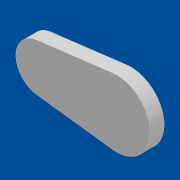
# Autodesk Inventor part: 111-base template
Saved by Autodesk Inventor 2018 (Build 220112000, 112)
## iProperties
Created: 2019-11-07
Part Number: 111-base template
Material: Generic
Document SubType Name: Modeling
Designer: Bunny320
Density: 1 g/cm^3
Appearance: Default
Author: Bunny320
Autodesk Inventor part; units mm, degrees
ref_plane "YZ Plane" through (0, 0, 0) normal (1, 0, 0) x (0, 1, 0)
ref_plane "XZ Plane" through (0, 0, 0) normal (0, 1, 0) x (-1, 0, 0)
ref_plane "XY Plane" through (0, 0, 0) normal (0, 0, 1) x (1, 0, 0)
sketch "Sketch2" plane through (0, 0, 0) normal (0, 1, 0) x (-1, 0, 0)
  circle A0 centre (0, 0) radius 40
  circle A1 centre (-141.8, 0) radius 57.5
  line L0 (4.9365, -39.6942) -> (-134.7037, -57.0604)
  line L1 (4.9365, 39.6942) -> (-134.7037, 57.0604)
  dimension "d5" = 141.8
  dimension "d6" = 80
  dimension "d7" = 115
  constraints: 4 end point, 4 point on circle, 4 tangent, 2 centre point, 1 coincident, 1 horizontal alignment
  measures "d5" distance of A1.centre point (0, 0)
  measures "d6" diameter of A0
  measures "d7" diameter of A1
extrude "Extrusion2" add sketch "Sketch2" along normal blind 4
sketch "Sketch14" plane through (0, 0, 0) normal (0, 1, 0) x (-1, 0, 0)
  arc A0 (4.9365, -39.6942) -> (4.9365, 39.6942) centre (0, 0) ccw projected
  arc A1 (5.4302, -43.6636) -> (5.4302, 43.6636) centre (0, 0) ccw
  arc A2 (-134.7037, 57.0604) -> (-134.7037, -57.0604) centre (-141.8, 0) ccw projected
  arc A3 (-134.2101, 61.0299) -> (-134.2101, -61.0299) centre (-141.8, 0) ccw
  line L0 (5.4302, -43.6636) -> (-134.2101, -61.0299)
  line L1 (-134.2101, 61.0299) -> (5.4302, 43.6636)
  line L2 (-134.7037, -57.0604) -> (4.9365, -39.6942)
  arc A4 (4.9365, -39.6942) -> (4.9365, 39.6942) centre (0, 0) ccw
  line L3 (4.9365, 39.6942) -> (-134.7037, 57.0604)
  arc A5 (-134.7037, 57.0604) -> (-134.7037, -57.0604) centre (-141.8, 0) ccw
  dimension "d53" = 4
  dimension "d54" = 4
  dimension "d55" = 4
  constraints: 8 end point, 8 point on circle, 4 centre point, 4 tangent, 2 coincident, 3 other
  measures "d53" radial gap between concentric circles of A0 A1
  measures "d54" radial gap between concentric circles of A2 A3
  measures "d55" distance between parallel lines of L2 L0
extrude "Extrusion11" add sketch "Sketch14" along normal blind 26
sketch "Sketch27" plane through (0, 4, 0) normal (0, 1, 0) x (1, 0, 0)
  line L0 (-40, 4) -> (-36, 4)
  line L1 (-36, 4) -> (-36, -4)
  line L2 (-36, -4) -> (-40, -4)
  line L3 (-40, -4) -> (-40, 4)
  line L4 (-40, 4) -> (-36, -4) construction
  line L5 (-36, 4) -> (-40, -4) construction
  arc A0 (-4.9365, 39.6942) -> (-4.9365, -39.6942) centre (0, 0) ccw projected
  line L6 (-4.9365, 39.6942) -> (134.7037, 57.0604) projected
  arc A1 (134.7037, -57.0604) -> (134.7037, 57.0604) centre (141.8, 0) ccw projected
  line L7 (195.3, 4) -> (199.3, 4)
  line L8 (199.3, 4) -> (199.3, -4)
  line L9 (199.3, -4) -> (195.3, -4)
  line L10 (195.3, -4) -> (195.3, 4)
  line L11 (195.3, 4) -> (199.3, -4) construction
  line L12 (199.3, 4) -> (195.3, -4) construction
  line L13 (134.7037, 57.0604) -> (-4.9365, 39.6942) projected
  line L14 (-4.9365, 39.6942) -> (3.0023, 40.6815)
  line L15 (3.0023, 40.6815) -> (3.4998, 36.6815)
  line L16 (3.4998, 36.6815) -> (-4.4391, 35.6942)
  line L17 (-4.4391, 35.6942) -> (-4.9365, 39.6942)
  line L18 (134.7037, -57.0604) -> (-4.9365, -39.6942) projected
  line L19 (-4.9365, -39.6942) -> (3.0023, -40.6815)
  line L20 (3.0023, -40.6815) -> (3.496, -36.7121)
  line L21 (3.496, -36.7121) -> (-4.4429, -35.7248)
  line L22 (-4.4429, -35.7248) -> (-4.9365, -39.6942)
  arc A2 (134.7037, -57.0604) -> (134.7037, 57.0604) centre (141.8, 0) ccw projected
  line L23 (134.7037, 57.0604) -> (126.7649, 56.0731)
  line L24 (126.7649, 56.0731) -> (127.2585, 52.1037)
  line L25 (127.2585, 52.1037) -> (135.1974, 53.091)
  line L26 (135.1974, 53.091) -> (134.7037, 57.0604)
  line L27 (134.7037, -57.0604) -> (126.7649, -56.0731)
  line L28 (126.7649, -56.0731) -> (127.2585, -52.1037)
  line L29 (127.2585, -52.1037) -> (135.1974, -53.091)
  line L30 (135.1974, -53.091) -> (134.7037, -57.0604)
  point P0 (-38, 0)
  point P1 (-38, 0)
  point P2 (-38, 0)
  point P3 (197.3, 0)
  point P4 (197.3, 0)
  dimension "d147" = 8
  dimension "d148" = 4
  dimension "d152" = 4
  dimension "d153" = 8
  dimension "d155" = 8
  dimension "d156" = 4
  dimension "d157" = 8
  dimension "d159" = 4
  dimension "d160" = 8
  dimension "d161" = 4
  dimension "d162" = 8
  dimension "d163" = 4
  constraints: 56 end point, 12 parallel, 6 midpoint, 6 perpendicular, 6 tangent, 4 point on line, 2 horizontal, 2 horizontal alignment, 1 coincident
  measures "d147" distance of L0.end L1.end
  measures "d148" distance of L1.end L2.end
  measures "d152" distance of L7.start L7.end
  measures "d153" distance of L9.end L7.start
  measures "d155" distance of L15.end L16.end
  measures "d156" vertical distance of L14.end L15.end
  measures "d157" distance of L20.end L21.end
  measures "d159" distance of L19.end L20.end
  measures "d160" distance of L24.end L25.end
  measures "d161" distance of L23.end L24.end
  measures "d162" distance of L28.end L29.end
  measures "d163" distance of L27.end L28.end
extrude "Extrusion19" add sketch "Sketch27" along normal up to surface (22 mm away) contours L0 A0 L3 | L0 L1 L2 A0 | A0 L2 L3 | L6 L15 L16 L17 | L22 L21 L20 L18 | L6 L26 L25 L24 | L28 L29 L30 L18 | L7 L8 A1 | A1 L9 L10 L7 | L8 L9 A1
fillet "Fillet4" radius 2 24 edges at (-39.7995, 15, -4) (-36, 15, -4) (-36, 15, 4) (-39.7995, 15, 4) (-4.9365, 15, -39.6942) (-4.4391, 15, -35.6942) (3.4998, 15, -36.6815) (3.0023, 15, -40.6815) (-4.9365, 15, 39.6942) (-4.4429, 15, 35.7248) (3.496, 15, 36.7121) (3.0023, 15, 40.6815) (127.2585, 15, -52.1037) (126.7649, 15, -56.0731) (134.7037, 15, -57.0604) (135.1974, 15, -53.091) (126.7649, 15, 56.0731) (127.2585, 15, 52.1037) (135.1974, 15, 53.091) (134.7037, 15, 57.0604) (199.1607, 15, -4) (195.3, 15, -4) (195.3, 15, 4) (199.1607, 15, 4)
sketch "Sketch28" plane through (0, 26, 0) normal (0, 1, 0) x (1, 0, 0)
  arc A0 (-4.9365, 39.6942) -> (-39.7995, 4) centre (0, 0) ccw projected
  line L0 (3.0023, 40.6815) -> (126.7649, 56.0731) projected
  arc A1 (199.1607, 4) -> (134.7037, 57.0604) centre (141.8, 0) ccw projected
  line L1 (126.7649, -56.0731) -> (3.0023, -40.6815) projected
  line L2 (3.0023, 40.6815) -> (3.4998, 36.6815) projected
  line L3 (127.2585, 52.1037) -> (126.7649, 56.0731) projected
  line L4 (3.496, -36.7121) -> (3.0023, -40.6815) projected
  line L5 (126.7649, -56.0731) -> (127.2585, -52.1037) projected
  point P0 (-40, 0)
  point P1 (-0.9671, 40.1879)
  point P2 (130.7343, 56.5668)
  point P3 (199.3, 0)
  point P4 (130.7343, -56.5668)
  point P5 (-0.9671, -40.1879)
  dimension "d164" = 4
  dimension "d165" = 4
  dimension "d166" = 4
  dimension "d167" = 4
  constraints: 4 point on line, 2 horizontal alignment, 2 point on circle
  measures "d164" distance from line of L2 point (-0.967, 40.188)
  measures "d165" distance from line of L3 point (130.734, 56.567)
  measures "d166" distance from line of L4 point (-0.967, -40.188)
  measures "d167" distance from line of L5 point (130.734, -56.567)
hole "Hole7" at (-40, 26, 0) at (-0.9671, 26, -40.1879) at (130.7343, 26, -56.5668) at (199.3, 26, 0) at (130.7343, 26, 56.5668) at (-0.9671, 26, 40.1879) direction (0, -1, 0) diameter 2.459 end through all thread size "M3x0.5" class "6H" standard "ISO Metric profile"
sketch "Sketch5" plane through (0, 4, 0) normal (0, 1, 0) x (1, 0, 0)
  arc A0 (134.7037, -57.0604) -> (134.7037, 57.0604) centre (141.8, 0) ccw projected
  circle A1 centre (141.8, 0) radius 45
  circle A2 centre (141.8, 0) radius 48
  point P0 (0, 0)
  dimension "d17" = 90
  dimension "d18" = 96
  constraints: 2 centre point, 2 coincident
  measures "d17" diameter of A1
  measures "d18" diameter of A2
sketch "Sketch6" plane through (141.8, 4, 0) normal (0, 1, 0) x (1, 0, 0)
  circle A0 centre (0, 0) radius 45 projected
  circle A1 centre (0, 0) radius 42
  point P0 (-141.8, 0)
  dimension "d146" = 84
  constraints: 1 centre point, 1 coincident
  measures "d146" diameter of A1
sketch "Sketch21" plane through (0, 4, 0) normal (0, 1, 0) x (1, 0, 0)
  line L0 (-25, 23) -> (25, 23) construction
  line L1 (-25, 21.3) -> (25, 21.3)
  line L2 (25, 24.7) -> (-25, 24.7)
  arc A0 (-25, 24.7) -> (-25, 21.3) centre (-25, 23) ccw
  arc A1 (25, 21.3) -> (25, 24.7) centre (25, 23) ccw
  point P0 (0, 0)
  point P1 (0, 23)
  dimension "d113" = 3.4
  dimension "d116" = 50
  dimension "d117" = 23
  constraints: 8 end point, 4 point on circle, 4 tangent, 2 centre point, 1 horizontal, 1 midpoint, 1 parallel, 1 vertical alignment
  measures "d113" distance between parallel lines of L2 L1
  measures "d116" distance of L0.start L0.end
  measures "d117" distance from line of point (0, 0) L0
sketch "Sketch22" plane through (0, 4, 0) normal (0, 1, 0) x (1, 0, 0)
  line L0 (-27, 29) -> (27, 29)
  line L1 (27, 29) -> (27, 26)
  line L2 (27, 26) -> (-27, 26)
  line L3 (-27, 26) -> (-27, 29)
  line L4 (-27, 29) -> (27, 26) construction
  line L5 (27, 29) -> (-27, 26) construction
  line L6 (-27, 20) -> (27, 20)
  line L7 (27, 20) -> (27, 17)
  line L8 (27, 17) -> (-27, 17)
  line L9 (-27, 17) -> (-27, 20)
  line L10 (-27, 20) -> (27, 17) construction
  line L11 (27, 20) -> (-27, 17) construction
  point P0 (0, 0)
  point P1 (0, 27.5)
  point P2 (0, 18.5)
  point P3 (0, 27.5)
  point P4 (0, 18.5)
  dimension "d148" = 4
  dimension "d118" = 6
  dimension "d119" = 3
  dimension "d120" = 3
  dimension "d121" = 26
  dimension "d122" = 54
  constraints: 24 end point, 6 midpoint, 4 parallel, 2 horizontal, 2 perpendicular, 2 vertical alignment, 1 point on line
  measures "d118" distance between parallel lines of L6 L2
  measures "d119" distance of L0.end L1.end
  measures "d120" distance of L6.end L7.end
  measures "d121" distance from line of point (0, 0) L2
  measures "d122" distance of L0.start L0.end
sketch "Sketch24" plane through (0, 4, 0) normal (0, 1, 0) x (1, 0, 0)
  line L0 (-27, -17.75) -> (27, -17.75)
  line L1 (27, -17.75) -> (27, 17.75)
  line L2 (27, 17.75) -> (-27, 17.75)
  line L3 (-27, 17.75) -> (-27, -17.75)
  line L4 (-27, -17.75) -> (27, 17.75) construction
  line L5 (27, -17.75) -> (-27, 17.75) construction
  point P0 (0, 0)
  dimension "d126" = 35.5
  dimension "d129" = 54
  constraints: 12 end point, 2 midpoint, 2 parallel, 1 horizontal, 1 perpendicular
  measures "d126" distance of L0.end L1.end
  measures "d129" distance of L1.end L2.end
equation "\"d53\" = d54"
equation "\"d55\" = d54"
equation "\"d155\" = d147"
equation "\"d156\" = d148"
equation "\"d157\" = d147"
equation "\"d159\" = d148"
equation "\"d160\" = d147"
equation "\"d161\" = d148"
equation "\"d162\" = d147"
equation "\"d163\" = d148"
equation "\"d164\" = d148"
equation "\"d165\" = d148"
equation "\"d166\" = d148"
equation "\"d167\" = d148"
equation "\"d120\" = d119"
equation "\"d121\" = d117 + 0.5 * d118"
body "Solid2"
